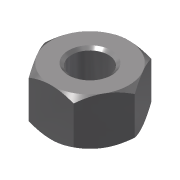
# Autodesk Inventor part: -
Saved by Autodesk Inventor 2021 (Build 250183000, 183)
## iProperties
Created: 2014-08-15
Part Number: -
Material: Stainless Steel
Document SubType Name: Modeling
Designer: dans
Mass: 90.098 g
Surface Area: 42.7185 cm^2
Volume: 11.1507 cm^3
Density: 8.08 g/cm^3
Appearance: Stainless - Brushed
Description: HEAVY HEX NUT-3/4"-10 UNC-ASTM A194 8M-SS
Author: dans
Autodesk Inventor part; units mm, degrees
ref_plane "YZ Plane" through (0, 0, 0) normal (1, 0, 0) x (0, 1, 0)
ref_plane "XZ Plane" through (0, 0, 0) normal (0, 1, 0) x (-1, 0, 0)
ref_plane "XY Plane" through (0, 0, 0) normal (0, 0, 1) x (1, 0, 0)
sketch "Sketch1" plane through (0, 0, 0) normal (0, 1, 0) x (-1, 0, 0)
  line L0 (9.1654, 15.875) -> (18.3309, 0)
  line L1 (18.3309, 0) -> (9.1654, -15.875)
  line L2 (9.1654, -15.875) -> (-9.1654, -15.875)
  line L3 (-9.1654, -15.875) -> (-18.3309, 0)
  line L4 (-18.3309, 0) -> (-9.1654, 15.875)
  line L5 (-9.1654, 15.875) -> (9.1654, 15.875)
  circle A0 centre (0, 0) radius 7.5
  dimension "HEX_FLATS" = 31.75
  dimension "NUT_SIZE" = 15
  constraints: 12 end point, 2 coincident, 1 centre point, 1 horizontal, 13 other
  measures "HEX_FLATS" distance between parallel lines of L2 L5
  measures "NUT_SIZE" diameter of A0
extrude "Extrusion1" add sketch "Sketch1" along normal mid plane 19.2532
sketch "Sketch2" plane through (0, 0, 0) normal (0, 0, 1) x (1, 0, 0)
  line L0 (18.3309, -9.6266) -> (9.1654, -9.6266) projected
  line L1 (15.875, -9.6266) -> (18.3309, -7.7216)
  line L2 (28.575, -7.7216) -> (28.575, -20.4216)
  line L3 (28.575, -20.4216) -> (15.875, -20.4216)
  line L4 (15.875, -20.4216) -> (15.875, -9.6266)
  line L5 (0, 0) -> (0, -1.2828)
  line L6 (18.3309, 9.6266) -> (18.3309, -9.6266) projected
  line L7 (18.3309, -7.7216) -> (28.575, -7.7216)
  line L8 (18.3309, 0) -> (27.089, 0) construction
  dimension "OUTSIDE_CHAMFER_LONG" = 15.875
  dimension "OUTSIDE_CHAMFER_SHORT" = 1.905
  dimension "d12" = 12.7
  dimension "d13" = 12.7
  constraints: 14 end point, 3 horizontal, 3 vertical, 2 point on line, 1 coincident, 1 midpoint
  measures "OUTSIDE_CHAMFER_LONG" distance from line of L4 L5.end
  measures "OUTSIDE_CHAMFER_SHORT" vertical distance of L1.start L1.end
  measures "d12" distance of L2.start L2.end
  measures "d13" distance of L2.end L3.end
revolve "Revolution1" cut sketch "Sketch2" angle 360 about axis through (0, 0, 0) along (0, -1, 0)
mirror "Mirror1" about plane through (0, 0, 0) normal (0, 1, 0) of "Revolution1"
chamfer "Chamfer1" distance 1.3208 angle 35 1 edges at (7.5, 9.6266, 0) measured on face at (8.9141, 9.6266, 9.4797)
chamfer "Chamfer2" distance 1.3208 angle 35 1 edges at (7.5, -9.6266, 0) measured on face at (8.9141, -9.6266, 9.4797)
body "Solid1"
